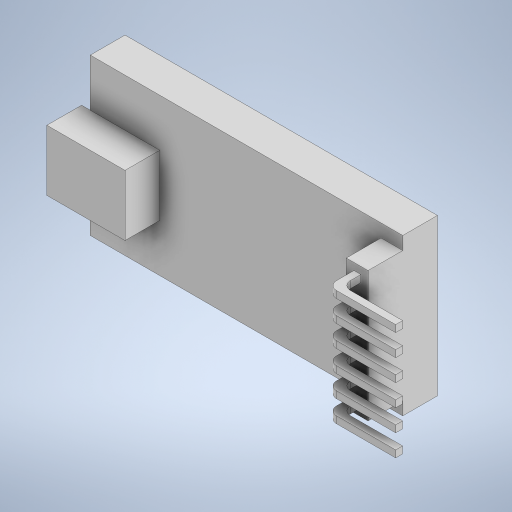
# Autodesk Inventor part: convertisseur
Saved by Autodesk Inventor 2024 (Build 280153000, 153)
## iProperties
Created: 2024-03-12
Part Number: convertisseur
Material: Générique
Document SubType Name: Modeling
Designer: phaly
Density: 1 g/cm^3
Appearance: Par défaut
Author: phaly
Autodesk Inventor part; units mm, degrees
ref_plane "YZ Plane" through (0, 0, 0) normal (1, 0, 0) x (0, 1, 0)
ref_plane "XZ Plane" through (0, 0, 0) normal (0, 1, 0) x (-1, 0, 0)
ref_plane "XY Plane" through (0, 0, 0) normal (0, 0, 1) x (1, 0, 0)
sketch "Esquisse1" plane through (0, 0, 0) normal (0, 0, 1) x (1, 0, 0)
  line L0 (0, 18) -> (36, 18)
  line L1 (36, 18) -> (36, 0)
  line L2 (36, 0) -> (0, 0)
  line L3 (0, 0) -> (0, 18)
  line L4 (-7.2, 0) -> (43.2, 0) projected
  line L5 (0, -3.6) -> (0, 21.6) projected
  point P0 (0, 0)
  dimension "d0" = 18
  dimension "d1" = 36
  constraints: 8 end point, 2 collinear, 2 parallel, 1 horizontal, 1 perpendicular
  measures "d0" distance of L2.end L0.start
  measures "d1" distance of L0.start L0.end
extrude "Extrusion1" add sketch "Esquisse1" along normal blind 4
sketch "Esquisse2" plane through (0, 0, 4) normal (0, 0, 1) x (1, 0, 0)
  line L0 (-1, 12.5) -> (8, 12.5)
  line L1 (8, 12.5) -> (8, 5.5)
  line L2 (8, 5.5) -> (-1, 5.5)
  line L3 (-1, 5.5) -> (-1, 12.5)
  line L4 (0, 0) -> (36, 0) projected
  line L5 (0, 18) -> (0, 0) projected
  dimension "d4" = 7
  dimension "d5" = 9
  dimension "d6" = 5.5
  dimension "d7" = 1
  constraints: 8 end point, 2 parallel, 1 horizontal, 1 perpendicular
  measures "d4" distance of L2.end L0.start
  measures "d5" distance of L0.start L0.end
  measures "d6" distance between parallel lines of L4 L2
  measures "d7" distance between parallel lines of L5 L3
extrude "Extrusion2" add sketch "Esquisse2" along normal blind 4
sketch "Esquisse3" plane through (0, 0, 4) normal (0, 0, 1) x (1, 0, 0)
  line L0 (33.5, 1.5) -> (36, 1.5)
  line L1 (36, 1.5) -> (36, 4)
  line L2 (36, 4) -> (33.5, 4)
  line L3 (33.5, 4) -> (33.5, 1.5)
  line L4 (36, 0) -> (36, 18) projected
  line L5 (33.5, 6.5) -> (33.5, 4)
  line L6 (36, 6.5) -> (33.5, 6.5)
  line L7 (36, 4) -> (36, 6.5)
  line L8 (33.5, 4) -> (36, 4)
  line L9 (33.5, 9) -> (33.5, 6.5)
  line L10 (36, 9) -> (33.5, 9)
  line L11 (36, 6.5) -> (36, 9)
  line L12 (33.5, 6.5) -> (36, 6.5)
  line L13 (33.5, 11.5) -> (33.5, 9)
  line L14 (36, 11.5) -> (33.5, 11.5)
  line L15 (36, 9) -> (36, 11.5)
  line L16 (33.5, 9) -> (36, 9)
  line L17 (33.5, 14) -> (33.5, 11.5)
  line L18 (36, 14) -> (33.5, 14)
  line L19 (36, 11.5) -> (36, 14)
  line L20 (33.5, 11.5) -> (36, 11.5)
  line L21 (33.5, 16.5) -> (33.5, 14)
  line L22 (36, 16.5) -> (33.5, 16.5)
  line L23 (36, 14) -> (36, 16.5)
  line L24 (33.5, 14) -> (36, 14)
  line L25 (0, 0) -> (36, 0) projected
  dimension "d10" = 2.5
  dimension "d11" = 2.5
  dimension "d14" = 2.5
  dimension "d19" = 1.5
  constraints: 48 end point, 2 parallel, 1 collinear, 1 horizontal, 1 perpendicular, 1 vertical, 40 other
  measures "d10" distance of L0.start L0.end
  measures "d11" distance of L2.end L0.start
  measures "d14" distance of L2.end L5.start
  measures "d19" distance between parallel lines of L25 L0
extrude "Extrusion3" add sketch "Esquisse3" along normal blind 4
sketch "Esquisse4" plane through (0, 0, 8) normal (0, 0, 1) x (1, 0, 0)
  line L0 (34.3859, 2.4) -> (35.1859, 2.4)
  line L1 (35.1859, 2.4) -> (35.1859, 3.2)
  line L2 (35.1859, 3.2) -> (34.3859, 3.2)
  line L3 (34.3859, 3.2) -> (34.3859, 2.4)
  line L4 (33.5, 16.5) -> (33.5, 1.5) projected
  line L5 (34.3859, 5.7) -> (34.3859, 4.9)
  line L6 (34.3859, 4.9) -> (35.1859, 4.9)
  line L7 (35.1859, 4.9) -> (35.1859, 5.7)
  line L8 (35.1859, 5.7) -> (34.3859, 5.7)
  line L9 (34.3859, 8.2) -> (34.3859, 7.4)
  line L10 (34.3859, 7.4) -> (35.1859, 7.4)
  line L11 (35.1859, 7.4) -> (35.1859, 8.2)
  line L12 (35.1859, 8.2) -> (34.3859, 8.2)
  line L13 (34.3859, 10.7) -> (34.3859, 9.9)
  line L14 (34.3859, 9.9) -> (35.1859, 9.9)
  line L15 (35.1859, 9.9) -> (35.1859, 10.7)
  line L16 (35.1859, 10.7) -> (34.3859, 10.7)
  line L17 (34.3859, 13.2) -> (34.3859, 12.4)
  line L18 (34.3859, 12.4) -> (35.1859, 12.4)
  line L19 (35.1859, 12.4) -> (35.1859, 13.2)
  line L20 (35.1859, 13.2) -> (34.3859, 13.2)
  line L21 (34.3859, 15.7) -> (34.3859, 14.9)
  line L22 (34.3859, 14.9) -> (35.1859, 14.9)
  line L23 (35.1859, 14.9) -> (35.1859, 15.7)
  line L24 (35.1859, 15.7) -> (34.3859, 15.7)
  line L25 (33.5, 1.5) -> (36, 1.5) projected
  point P0 (0, 0)
  dimension "d22" = 0.8
  dimension "d23" = 0.8
  dimension "d26" = 2.5
  dimension "d31" = 0.9
  constraints: 48 end point, 2 parallel, 1 horizontal, 1 perpendicular, 1 vertical, 40 other
  measures "d22" distance of L2.end L0.start
  measures "d23" distance of L0.start L0.end
  measures "d26" distance of L2.end L5.start
  measures "d31" distance between parallel lines of L25 L0
extrude "Extrusion4" add sketch "Esquisse4" along normal blind 3
sketch "Esquisse5" plane through (35.1859, 14.9, 8) normal (1, 0, 0) x (0, 0, -1)
  line L0 (-3, 0) -> (-3, 0.8) projected
  line L1 (-3, 0.8) -> (-2.2, 0.8)
  line L2 (-2.2, 0.8) -> (-2.2, 0)
  line L3 (-2.2, 0) -> (-3, 0)
  line L4 (-3, 0) -> (-3, 0.8)
  line L5 (0, 0) -> (-3, 0) projected
  line L6 (0, -13.4) -> (0, 1.6) projected
  line L7 (-2.2, -1.7) -> (-2.2, -2.5)
  line L8 (-3, -1.7) -> (-2.2, -1.7)
  line L9 (-3, -2.5) -> (-3, -1.7)
  line L10 (-2.2, -2.5) -> (-3, -2.5)
  line L11 (-2.2, -4.2) -> (-2.2, -5)
  line L12 (-3, -4.2) -> (-2.2, -4.2)
  line L13 (-3, -5) -> (-3, -4.2)
  line L14 (-2.2, -5) -> (-3, -5)
  line L15 (-2.2, -6.7) -> (-2.2, -7.5)
  line L16 (-3, -6.7) -> (-2.2, -6.7)
  line L17 (-3, -7.5) -> (-3, -6.7)
  line L18 (-2.2, -7.5) -> (-3, -7.5)
  line L19 (-2.2, -9.2) -> (-2.2, -10)
  line L20 (-3, -9.2) -> (-2.2, -9.2)
  line L21 (-3, -10) -> (-3, -9.2)
  line L22 (-2.2, -10) -> (-3, -10)
  line L23 (-2.2, -11.7) -> (-2.2, -12.5)
  line L24 (-3, -11.7) -> (-2.2, -11.7)
  line L25 (-3, -12.5) -> (-3, -11.7)
  line L26 (-2.2, -12.5) -> (-3, -12.5)
  point P0 (8, -14.9)
  dimension "d34" = 0.8
  dimension "d37" = 2.5
  constraints: 48 end point, 2 parallel, 1 collinear, 1 horizontal, 1 perpendicular, 1 vertical, 40 other
  measures "d34" distance of L2.end L3.end
  measures "d37" distance of L1.end L7.start
extrude "Extrusion5" add sketch "Esquisse5" along normal blind 7
fillet "Congé1" radius 1 12 edges at (34.3859, 15.3, 11) (34.3859, 12.8, 11) (34.3859, 10.3, 11) (34.3859, 7.8, 11) (34.3859, 5.3, 11) (34.3859, 2.8, 11) (35.1859, 2.8, 10.2) (35.1859, 5.3, 10.2) (35.1859, 7.8, 10.2) (35.1859, 10.3, 10.2) (35.1859, 12.8, 10.2) (35.1859, 15.3, 10.2)
equation "\"d23\" = d22"
